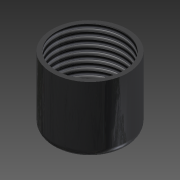
# Autodesk Inventor part: Nakrętka_wentyla
Saved by Autodesk Inventor 2015 (Build 190159000, 159)
## iProperties
Created: 2016-01-13
Part Number: Nakrętka_wentyla
Material: Kauczuk
Document SubType Name: Modeling
Designer: graaapsik
Density: 0.93 g/cm^3
Appearance: Kauczuk - czarny - wersja 1.1
Mass: 0.117348 g
Surface Area: 5.29344 cm^2
Volume: 0.12618 cm^3
Author: graaapsik
Autodesk Inventor part; units mm, degrees
ref_plane "YZ Plane" through (0, 0, 0) normal (1, 0, 0) x (0, 1, 0)
ref_plane "XZ Plane" through (0, 0, 0) normal (0, 1, 0) x (-1, 0, 0)
ref_plane "XY Plane" through (0, 0, 0) normal (0, 0, 1) x (1, 0, 0)
sketch "Szkic1" plane through (0, 0, 0) normal (0, 0, 1) x (1, 0, 0)
  circle A0 centre (0, 0) radius 4.5
  dimension "d0" = 9
  constraints: 1 centre point, 1 coincident
  measures "d0" diameter of A0
extrude "Wyciągnięcie proste1" add sketch "Szkic1" along normal blind 8
shell "Skorupa1" thickness 0.5 removed faces 1 at (0.1808, 1.316, 8)
thread "Gwint1" size "M8x0.8" class "6H" standard "ANSI Metric M Profile" full length
fillet "Zaokrąglenie1" radius 1 1 edges at (-4.5, 0, 0)
